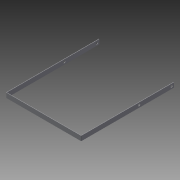
# Autodesk Inventor part: 4barRoundedBar
Saved by Autodesk Inventor 2015 SP1 (Build 190203100, 203)
## iProperties
Created: 2015-02-16
Part Number: 4barRoundedBar
Material: Generic
Document SubType Name: Modeling
Designer: 55221
Density: 1 g/cm^3
Appearance: Default
Author: 55221
Autodesk Inventor part; units mm, degrees
ref_plane "YZ Plane" through (0, 0, 0) normal (1, 0, 0) x (0, 1, 0)
ref_plane "XZ Plane" through (0, 0, 0) normal (0, 1, 0) x (-1, 0, 0)
ref_plane "XY Plane" through (0, 0, 0) normal (0, 0, 1) x (1, 0, 0)
sketch "Sketch1" plane through (0, 0, 0) normal (0, 1, 0) x (-1, 0, 0)
  line L0 (406.4, 508) -> (0, 508)
  line L1 (0, 508) -> (0, 0)
  line L2 (406.4, 0) -> (406.4, 508)
  line L3 (408.94, 505.46) -> (-2.54, 505.46)
  line L4 (-2.54, 505.46) -> (-2.54, 0)
  line L5 (408.94, 0) -> (408.94, 505.46)
  arc A0 (408.94, 505.46) -> (406.4, 508) centre (406.4, 505.46) ccw
  arc A1 (0, 508) -> (-2.54, 505.46) centre (0, 505.46) ccw
  line L6 (0, 505.46) -> (0, 0)
  line L7 (408.94, 0) -> (406.4, 0)
  line L8 (0, 0) -> (-2.54, 0)
  dimension "d0" = 411.48
  dimension "d1" = 2.54
  constraints: 18 end point, 4 point on circle, 3 equal length, 3 horizontal, 2 centre point, 2 perpendicular, 2 tangent
  measures "d0" distance of L5.start L4.end
  measures "d1" radius of A1
extrude "Extrusion1" add sketch "Sketch1" against normal blind 25.4
sketch "Sketch2" plane through (2.54, 0, 505.46) normal (1, 0, 0) x (0, 0, -1)
  circle A0 centre (492.76, -12.7) radius 6.35
  point P0 (505.46, 0)
  dimension "d4" = 12.7
  constraints: 1 centre point
  measures "d4" diameter of A0
extrude "Extrusion2" cut sketch "Sketch2" against normal blind 411.48
sketch "Sketch3" plane through (2.54, 0, 505.46) normal (1, 0, 0) x (0, 0, -1)
  circle A0 centre (314.96, -12.7) radius 6.35
  point P0 (505.46, 0)
  dimension "d7" = 12.7
  constraints: 1 centre point
  measures "d7" diameter of A0
extrude "Extrusion3" cut sketch "Sketch3" against normal blind 411.48
body "Solid1"
